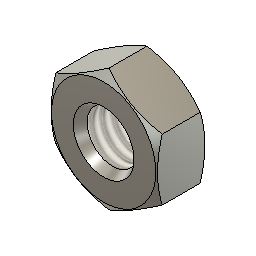
y mount v18 (Autodesk Fusion 360 archive; units mm, degrees)
design "Hexagon Regular Nut SS-EN ISO 4032 - M4 Steel 6 Plain"
description: Hexagon Regular Nut SS-EN ISO 4032 - M4
Autodesk Fusion 360 part; units mm, degrees
sketch "Sketch1" plane through (0, 0, 0) normal (0, 1, 0) x (1, 0, 0)
  line L0 (0, 0) -> (0, -3.2)
  line L1 (-2, 0) -> (-3.43, 0)
  line L2 (-3.43, 0) -> (-4.0425, -0.3536)
  line L3 (-4.0425, -0.3536) -> (-4.0425, -2.8464)
  line L4 (-4.0425, -2.8464) -> (-3.43, -3.2)
  line L5 (-3.43, -3.2) -> (-2, -3.2)
  line L6 (-2, -3.2) -> (-2, 0)
  dimension "d121" = 4
  dimension "d122" = 30
  dimension "d123" = 30
  dimension "d126" = 3.2
  dimension "d128" = 8.085
  dimension "d172" = 6.86
  constraint vertical L0
  constraint coincident L0 L0.end
  constraint coincident origin L0
  constraint horizontal L1
  constraint perpendicular L1 L3
  constraint perpendicular L3 L5
  constraint perpendicular L5 L6
  constraint coincident L0.start L1
  constraint coincident L0.start origin
  constraint coincident L0.end L5
  constraint equal L1 L5
  measures "d122" angle of L1 L2
  measures "d123" angle of L4 L5
  measures "d126" distance of L1.start L5.end
revolve "Revolve1" add sketch "Sketch1" angle 360 about axis through (0, 0, 0) along (0, 0, 1)
sketch "Sketch8" plane through (0, 0, 3.2) normal (0, 0, 1) x (1, 0, 0)
  line L0 (0, 0) -> (-7, 0) construction
  line L1 (-3.5, -2.0228) -> (-3.5, 2.0228)
  circle A0 centre (0, 0) radius 2
  circle A1 centre (0, 0) radius 4.0425
  dimension "d114" = 3.5
  constraint horizontal L0
  constraint perpendicular L0 L1
  constraint midpoint L0 L1
  constraint coincident L0.start A0.centre
  constraint coincident L1.end A1
  measures "d114" distance of L0.start L1
extrude "Extrude5" cut sketch "Sketch8" against normal blind 3.2 contours L1 A1 picked at (-3.5875, -0.4927)
pattern_circular "C-Pattern2" count 6 over 360 about axis through (0, 0, 1.75) along (0, 0, 1) of "Extrude5"
thread "Thread3" "ISO Metric profile 4.0 M4x0.7 6H" major diameter 4.1095 minor diameter 3.332 pitch 0.7 angle 60 resizes the face on face at (-1.9975, 0.0997, 2.1333)
sketch "Sketch12" plane through (0, 0, 0) normal (0, 1, 0) x (1, 0, 0)
  line L0 (1.666, -3.2) -> (-1.666, -3.2)
  line L1 (3.43, -3.2) -> (-3.43, -3.2)
  line L2 (3.43, 0) -> (-3.43, 0)
  line L3 (1.666, 0) -> (-1.666, 0)
  line L4 (-2, 0) -> (0, 0)
  line L5 (-1.0762, -1.6) -> (-2, 0)
  line L6 (-2, -3.2) -> (0, -3.2)
  line L7 (-1.0762, -1.6) -> (-2, -3.2)
  line L8 (0, 0) -> (0, -3.2)
  dimension "d165" = 60
  dimension "d169" = 60
  dimension "d170" = 2
  constraint horizontal L4
  constraint collinear L1 L6
  constraint coincident L5.start L7.start
  constraint vertical L4.start L6.start
  constraint coincident L1 L6.end
  constraint coincident L6.end L8.end
  constraint coincident L4.end L8.start
  measures "d165" angle of L2 L5
  measures "d169" angle of L6 L7
  measures "d170" distance of L4.start L4.end
revolve "Revolve3" cut sketch "Sketch12" angle 360 about axis through (0, 0, 1.75) along (0, 0, 1)
equation "adsk_nheig = 3.20 mm"
equation "adsk_maxdia = 8.085 mm"
equation "adsk_nomdia = 4.00 mm"
equation "d89 = -adsk_nheig"
equation "adsk_waflat = 7.00 mm"
equation "d114 = adsk_waflat / 2"
equation "adsk_chamang1 = 30.00 deg"
equation "adsk_chamang2 = 30.00 deg"
equation "d121 = adsk_nomdia"
equation "d122 = adsk_chamang1"
equation "d123 = adsk_chamang2"
equation "d126 = adsk_nheig"
equation "d128 = adsk_maxdia"
equation "d163 = adsk_nheig"
equation "d170 = adsk_nomdia * 0.5"
equation "adsk_beardia = adsk_waflat * 0.98"
equation "d172 = adsk_beardia"

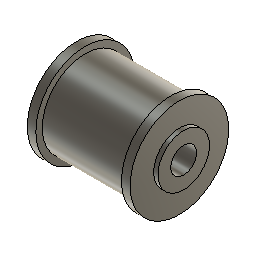
design "f623 bearing stack 9mm"
Autodesk Fusion 360 part; units mm, degrees
sketch "Sketch1" plane through (0, 0, 0) normal (1, 0, 0) x (0, 1, 0)
  circle A0 centre (0, 0) radius 5
  circle A1 centre (0, 0) radius 5.75
  circle A2 centre (0, 0) radius 1.5
  dimension "d1" = 10
  dimension "d2" = 11.5
  dimension "d3" = 3
  constraint coincident A0.centre A1.centre
  constraint concentric A0 A2
  measures "d1" diameter of A0
  measures "d2" diameter of A1
  measures "d3" diameter of A2
extrude "Extrude1" add sketch "Sketch1" along normal mid plane 12 contours A0
extrude "Extrude2" add sketch "Sketch1" against normal blind 1 from surface at 6 contours A1
mirror "Mirror1" about plane through (0, 0, 0) normal (1, 0, 0) of "Extrude2"
sketch "Sketch2" plane through (-6, 0, 0) normal (-1, 0, 0) x (0, -1, 0)
  circle A0 centre (0, 0) radius 5.75
  circle A1 centre (0, 0) radius 1.5
  circle A2 centre (0, 0) radius 3
  dimension "d11" = 6
  constraint coincident A0.centre A1.centre
  measures "d11" diameter of A2
extrude "Extrude3" add sketch "Sketch2" along normal blind 0.5 contours A2
mirror "Mirror2" about plane through (0, 0, 0) normal (1, 0, 0) of "Extrude3"
equation "d4 = ( 4 * 3 ) * 1 mm"

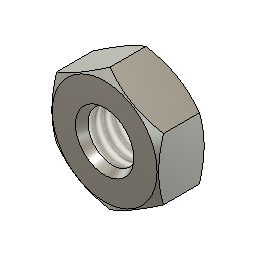
design "Hexagon Regular Nut ISO 4032 - M3 Steel 6 Plain"
description: Hexagon Regular Nut ISO 4032 - M3
Autodesk Fusion 360 part; units mm, degrees
sketch "Sketch1" plane through (0, 0, 0) normal (0, 1, 0) x (1, 0, 0)
  line L0 (0, 0) -> (0, -2.4)
  line L1 (-1.5, 0) -> (-2.695, 0)
  line L2 (-2.695, 0) -> (-3.1763, -0.2778)
  line L3 (-3.1763, -0.2778) -> (-3.1763, -2.1222)
  line L4 (-3.1763, -2.1222) -> (-2.695, -2.4)
  line L5 (-2.695, -2.4) -> (-1.5, -2.4)
  line L6 (-1.5, -2.4) -> (-1.5, 0)
  dimension "d121" = 3
  dimension "d122" = 30
  dimension "d123" = 30
  dimension "d126" = 2.4
  dimension "d128" = 6.3525
  dimension "d172" = 5.39
  constraint vertical L0
  constraint coincident L0 L0.end
  constraint coincident origin L0
  constraint horizontal L1
  constraint perpendicular L1 L3
  constraint perpendicular L3 L5
  constraint perpendicular L5 L6
  constraint coincident L0.start L1
  constraint coincident L0.start origin
  constraint coincident L0.end L5
  constraint equal L1 L5
  measures "d122" angle of L1 L2
  measures "d123" angle of L4 L5
  measures "d126" distance of L1.start L5.end
revolve "Revolve1" add sketch "Sketch1" angle 360 about axis through (0, 0, 0) along (0, 0, 1)
sketch "Sketch8" plane through (0, 0, 2.4) normal (0, 0, 1) x (1, 0, 0)
  line L0 (0, 0) -> (-5.5, 0) construction
  line L1 (-2.75, -1.5894) -> (-2.75, 1.5894)
  circle A0 centre (0, 0) radius 1.5
  circle A1 centre (0, 0) radius 3.1763
  dimension "d114" = 2.75
  constraint horizontal L0
  constraint perpendicular L0 L1
  constraint midpoint L0 L1
  constraint coincident L0.start A0.centre
  constraint coincident L1.end A1
  measures "d114" distance of L0.start L1
extrude "Extrude5" cut sketch "Sketch8" against normal blind 2.4 contours L1 A1 picked at (-2.8188, 0.3871)
pattern_circular "C-Pattern2" count 6 over 360 about axis through (0, 0, 1.75) along (0, 0, 1) of "Extrude5"
thread "Thread3" "ISO Metric profile 3.0 M3x0.5 6H" major diameter 3.086 minor diameter 2.529 pitch 0.5 angle 60 resizes the face on face at (-1.4925, 0.1494, 1.6)
sketch "Sketch12" plane through (0, 0, 0) normal (0, 1, 0) x (1, 0, 0)
  line L0 (1.2645, -2.4) -> (-1.2645, -2.4)
  line L1 (2.695, -2.4) -> (-2.695, -2.4)
  line L2 (2.695, 0) -> (-2.695, 0)
  line L3 (1.2645, 0) -> (-1.2645, 0)
  line L4 (-1.5, 0) -> (0, 0)
  line L5 (-0.8072, -1.2) -> (-1.5, 0)
  line L6 (-1.5, -2.4) -> (0, -2.4)
  line L7 (-0.8072, -1.2) -> (-1.5, -2.4)
  line L8 (0, 0) -> (0, -2.4)
  dimension "d165" = 60
  dimension "d169" = 60
  dimension "d170" = 1.5
  constraint horizontal L4
  constraint collinear L1 L6
  constraint coincident L5.start L7.start
  constraint vertical L4.start L6.start
  constraint coincident L1 L6.end
  constraint coincident L6.end L8.end
  constraint coincident L4.end L8.start
  measures "d165" angle of L2 L5
  measures "d169" angle of L6 L7
  measures "d170" distance of L4.start L4.end
revolve "Revolve3" cut sketch "Sketch12" angle 360 about axis through (0, 0, 1.75) along (0, 0, 1)
equation "adsk_nheig = 2.40 mm"
equation "adsk_maxdia = 6.3525 mm"
equation "adsk_nomdia = 3.00 mm"
equation "d89 = -adsk_nheig"
equation "adsk_waflat = 5.50 mm"
equation "d114 = adsk_waflat / 2"
equation "adsk_chamang1 = 30.00 deg"
equation "adsk_chamang2 = 30.00 deg"
equation "d121 = adsk_nomdia"
equation "d122 = adsk_chamang1"
equation "d123 = adsk_chamang2"
equation "d126 = adsk_nheig"
equation "d128 = adsk_maxdia"
equation "d163 = adsk_nheig"
equation "d170 = adsk_nomdia * 0.5"
equation "adsk_beardia = adsk_waflat * 0.98"
equation "d172 = adsk_beardia"
